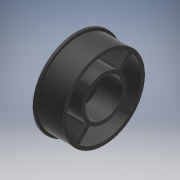
# Autodesk Inventor part: 바퀴
Saved by Autodesk Inventor 2017 (Build 210142000, 142)
## iProperties
Part Number: 바퀴
Material: 아세탈 수지, 검은색
Document SubType Name: Modeling
Designer: minom
Density: 1.425 g/cm^3
Appearance: 매끄러움 - 검은색
Mass: 59.5415 g
Surface Area: 234.199 cm^2
Volume: 41.7835 cm^3
Author: minom
Autodesk Inventor part; units mm, degrees
ref_plane "YZ Plane" through (0, 0, 0) normal (1, 0, 0) x (0, 1, 0)
ref_plane "XZ Plane" through (0, 0, 0) normal (0, 1, 0) x (-1, 0, 0)
ref_plane "XY Plane" through (0, 0, 0) normal (0, 0, 1) x (1, 0, 0)
sketch "스케치1" plane through (0, 0, 0) normal (1, 0, 0) x (0, 1, 0)
  circle A0 centre (0, 0) radius 37
  dimension "d0" = 74
  constraints: 1 centre point, 1 coincident
  measures "d0" diameter of A0
extrude "돌출1" add sketch "스케치1" along normal blind 24
sketch "스케치2" plane through (24, 0, 0) normal (1, 0, 0) x (0, 0, -1)
  circle A0 centre (0, 0) radius 5
  dimension "d3" = 10
  constraints: 1 centre point, 1 coincident
  measures "d3" diameter of A0
extrude "돌출2" cut sketch "스케치2" against normal blind 24
sketch "스케치3" plane through (24, 0, 0) normal (1, 0, 0) x (0, 0, -1)
  circle A0 centre (0, 0) radius 5
  circle A1 centre (0, 0) radius 16
  constraints: 2 centre point, 1 coincident
extrude "돌출4" cut sketch "스케치3" against normal blind 19
sketch "스케치4" plane through (5, 0, 0) normal (1, 0, 0) x (0, 0, -1)
  circle A0 centre (-10, 0) radius 1.75
  circle A1 centre (0, 10) radius 1.75
  circle A2 centre (10, 0) radius 1.75
  circle A3 centre (0, -10) radius 1.75
  point P0 (0, 0)
  dimension "d21" = 3.5
  dimension "d22" = 3.5
  dimension "d23" = 3.5
  dimension "d24" = 3.5
  constraints: 4 centre point
  measures "d21" diameter of A0
  measures "d22" diameter of A1
  measures "d23" diameter of A2
  measures "d24" diameter of A3
extrude "돌출5" cut sketch "스케치4" against normal blind 19
sketch "스케치5" plane through (24, 0, 0) normal (1, 0, 0) x (0, 0, -1)
  circle A0 centre (0, 0) radius 19
  circle A1 centre (0, 0) radius 32
  line L0 (0, 0) -> (-22.6274, 22.6274)
  line L1 (0, 0) -> (32, 0) construction
  line L2 (-22.6274, 22.6274) -> (22.6274, -22.6274)
  line L3 (0, 0) -> (-22.6274, -22.6274)
  line L4 (0, 0) -> (32, 0) construction
  line L5 (-22.6274, -22.6274) -> (22.6274, 22.6274)
  line L6 (-18, 18) -> (-16.5858, 19.4142)
  line L7 (-16.5858, 19.4142) -> (-19.4142, 16.5858)
  line L8 (-16.5858, 19.4142) -> (-11.9462, 14.7746)
  line L9 (-21.169, 23.9974) -> (-16.5858, 19.4142)
  line L10 (-19.4142, 16.5858) -> (-23.9974, 21.169)
  line L11 (-14.7746, 11.9462) -> (-19.4142, 16.5858)
  line L12 (18, 18) -> (16.5858, 19.4142)
  line L13 (16.5858, 19.4142) -> (19.4142, 16.5858)
  line L14 (19.4142, 16.5858) -> (14.7746, 11.9462)
  line L15 (23.9974, 21.169) -> (19.4142, 16.5858)
  line L16 (16.5858, 19.4142) -> (21.169, 23.9974)
  line L17 (16.5858, 19.4142) -> (11.9462, 14.7746)
  line L18 (18, -18) -> (19.4142, -16.5858)
  line L19 (19.4142, -16.5858) -> (16.5858, -19.4142)
  line L20 (16.5858, -19.4142) -> (11.9462, -14.7746)
  line L21 (16.5858, -19.4142) -> (21.169, -23.9974)
  line L22 (19.4142, -16.5858) -> (14.7746, -11.9462)
  line L23 (19.4142, -16.5858) -> (23.9974, -21.169)
  line L24 (-18, -18) -> (-19.4142, -16.5858)
  line L25 (-19.4142, -16.5858) -> (-16.5858, -19.4142)
  line L26 (-16.5858, -19.4142) -> (-11.9462, -14.7746)
  line L27 (-16.5858, -19.4142) -> (-21.169, -23.9974)
  line L28 (-19.4142, -16.5858) -> (-14.7746, -11.9462)
  line L29 (-23.9974, -21.169) -> (-19.4142, -16.5858)
  dimension "d27" = 38
  dimension "d28" = 64
  dimension "d29" = 135
  dimension "d30" = 135
  dimension "d31" = 2
  dimension "d32" = 4
  dimension "d33" = 2
  constraints: 60 end point, 22 point on line, 6 perpendicular, 4 parallel, 3 collinear, 2 coincident, 2 equal length, 2 horizontal, 24 other
  measures "d29" angle of L1 L0
  measures "d30" angle of L3 L4
  measures "d31" distance of L6.start L6.end
  measures "d32" distance of L6.end L7.end
  measures "d33" distance of L12.start L12.end
extrude "돌출6" cut sketch "스케치5" against normal blind 19 contours A0 L14 L15 A1 L23 L22 | A0 L8 L9 A1 L16 L17 | L20 L21 A1 L27 L26 A0 | A0 L28 L29 A1 L10 L11
sketch "스케치6" plane through (24, 0, 0) normal (1, 0, 0) x (0, 0, -1)
  circle A0 centre (0, 0) radius 35
  circle A1 centre (0, 0) radius 37
  dimension "d36" = 70
  dimension "d37" = 74
  constraints: 2 centre point, 2 coincident
  measures "d36" diameter of A0
  measures "d37" diameter of A1
extrude "돌출7" cut sketch "스케치6" against normal blind 22
